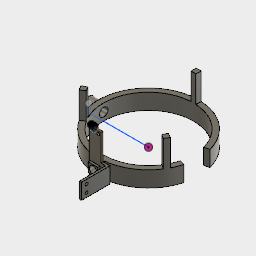
500 ml band v12 (Autodesk Fusion 360 design; units mm, degrees)
Autodesk Fusion 360 part; units mm, degrees
note: some values were not read from the file. Set by a fixed rule: which sketch regions a step uses.
sketch "Sketch1" plane through (0, 0, 0) normal (0, 1, 0) x (1, 0, 0)
  circle A0 centre (0, 0) radius 42.5
  circle A1 centre (0, 0) radius 47.5
  dimension "d1" = 85
  dimension "d2" = 5
  measures "d1" diameter of A0
extrude "Extrude1" add sketch "Sketch1" along normal blind 15
sketch "Sketch2" plane through (0, 15, 0) normal (0, 1, 0) x (-1, 0, 0)
  circle A0 centre (0, 0) radius 42.5
  circle A1 centre (0, 0) radius 47.5
  line L0 (0, 0) -> (2.4844, -47.435)
  line L1 (0, 0) -> (-2.5267, -47.4328)
extrude "Extrude2" add sketch "Sketch2" along normal blind 25 contours A0 A1 L0 L1 picked at (1.3425, -45.8073)
sketch "Sketch3" plane through (0, 15, 0) normal (0, 1, 0) x (-1, 0, 0)
  line L0 (2.2229, -42.4418) -> (2.4844, -47.435)
  arc A0 (2.4844, -47.435) -> (-2.5267, -47.4328) centre (0, 0) ccw
  line L1 (-2.5267, -47.4328) -> (-2.2607, -42.4398)
  arc A1 (2.2229, -42.4418) -> (-2.2607, -42.4398) centre (0, 0) ccw
  line L2 (0, 0) -> (42.3334, 21.5437)
  line L3 (0, 0) -> (39.8389, 25.8672)
extrude "Extrude3" add sketch "Sketch3" along normal blind 25 contours A0 A1 L2 L3
sketch "Sketch4" plane through (0, 15, 0) normal (0, 1, 0) x (-1, 0, 0)
  line L0 (35.6453, 23.1443) -> (39.8389, 25.8672)
  arc A0 (39.8389, 25.8672) -> (-2.5267, -47.4328) centre (0, 0) ccw
  line L1 (-2.5267, -47.4328) -> (-2.2607, -42.4398)
  arc A1 (35.6453, 23.1443) -> (-2.2607, -42.4398) centre (0, 0) ccw
  line L2 (0, 0) -> (-39.8369, 25.8704)
  line L3 (0, 0) -> (47.5, 0) construction
  line L4 (0, 0) -> (-42.3228, 21.5645)
  line L5 (0, 0) -> (47.5, 0) construction
  dimension "d9" = 147
  dimension "d10" = 47.5
  dimension "d11" = 153
  dimension "d12" = 47.5
  measures "d9" angle of L2 L3
  measures "d10" distance of A0.centre L2.end
  measures "d11" angle of L4 L5
  measures "d12" distance of A0.centre L4.end
extrude "Extrude4" add sketch "Sketch4" along normal blind 25 contours A0 A1 L2 L4
sketch "Sketch5" plane through (0, 15, 0) normal (0, 1, 0) x (-1, 0, 0)
  line L0 (-37.8678, 19.2946) -> (-42.3228, 21.5645)
  arc A0 (-42.3228, 21.5645) -> (-2.5267, -47.4328) centre (0, 0) ccw
  line L1 (-2.5267, -47.4328) -> (-2.2607, -42.4398)
  arc A1 (-37.8678, 19.2946) -> (-2.2607, -42.4398) centre (0, 0) ccw
  line L2 (0, 0) -> (-45.8815, 12.2939)
  line L3 (0, 0) -> (47.5, 0) construction
  line L4 (0, 0) -> (-45.8815, -12.2939)
  line L5 (0, 0) -> (47.5, 0) construction
  dimension "d15" = 165
  dimension "d16" = 47.5
  dimension "d17" = 165
  dimension "d18" = 47.5
  measures "d15" angle of L2 L3
  measures "d16" distance of A0.centre L2.end
  measures "d17" angle of L4 L5
  measures "d18" distance of A0.centre L4.end
extrude "Extrude5" cut sketch "Sketch5" against normal blind 15 contours A0 A1 L2 L4
sketch "Sketch6" plane through (0, 0, 0) normal (0, 0, 1) x (1, 0, 0)
  line L0 (0, 0) -> (5.5, 0)
  line L1 (5.5, 0) -> (5.5, 2)
  line L2 (5.5, 2) -> (-5.5, 2)
  line L3 (-5.5, 2) -> (-5.5, 13)
  line L4 (-5.5, 13) -> (5.5, 13)
  line L5 (5.5, 13) -> (5.5, 2)
  dimension "d21" = 5.5
  dimension "d22" = 2
  dimension "d23" = 11
  dimension "d24" = 11
  measures "d21" distance of L0.start L0.end
  measures "d22" distance of L0.end L1.end
  measures "d23" distance of L1.end L2.end
  measures "d24" distance of L1.end L4.end
extrude "Extrude6" cut sketch "Sketch6" along normal blind 50
sketch "Sketch8" plane through (0, 0, 0) normal (0, 0, 1) x (1, 0, 0)
  line L0 (0, 0) -> (-56.7, 0)
  line L1 (-56.7, 0) -> (-56.7, 7.5)
  dimension "d28" = 56.7
  dimension "d29" = 7.5
  measures "d28" distance of L0.start L0.end
  measures "d29" distance of L0.end L1.end
sketch "Sketch9" plane through (0, 0, 0) normal (1, 0, 0) x (0, 0, -1)
  point P0 (0, 7.5)
ref_plane "WorkPlane1" through (-56.7, 7.5, 0) normal (1, 0, 0) x (0, 0, -1)
cylinder "CylinderPrimitive1" add diameter 12 height 14.2 placed x (0, 0, -1) y (0, 1, 0) z (1, 0, 0) at (-56.7, 7.5, 0)
hole "Hole1" at (-56.7, 7.5, 0) direction (1, 0, 0) diameter 6.8 depth 2.2 tip angle 180
sketch "Sketch11" plane through (0, 0, 0) normal (1, 0, 0) x (0, 0, -1)
  circle A0 centre (0, 7.5) radius 4
  point P0 (0, 7.5)
  dimension "d37" = 8
  measures "d37" diameter of A0
extrude "Extrude7" cut sketch "Sketch11" against normal blind 54.5
sketch "Sketch16" plane through (0, 0, 0) normal (0, 1, 0) x (1, 0, 0)
extrude "Extrude13" add sketch "Sketch6" along normal blind 50.5
move_face "OffsetFaces2" offset -42.5 1 faces at (1.8333, 5.6667, 0)
sketch "Sketch17" plane through (0, 0, 50.5) normal (0, 0, 1) x (1, 0, 0)
  line L0 (5.5, 13) -> (-5.5, 13)
  line L1 (-5.5, 13) -> (-5.5, 2)
  line L2 (-5.5, 2) -> (5.5, 2)
  line L3 (5.5, 2) -> (5.5, 13)
  line L4 (-4.5, 12) -> (-4.5, 3)
  line L5 (-4.5, 3) -> (4.5, 3)
  line L6 (4.5, 3) -> (4.5, 12)
  line L7 (4.5, 12) -> (-4.5, 12)
  dimension "d60" = 1
extrude "Extrude14" add sketch "Sketch17" along normal blind 2 contours L4 L5 L6 L7
move_face "OffsetFaces3" offset 2 1 faces at (-0.6123, 13, 49.4882)
move_face "OffsetFaces4" offset 2 1 faces at (-0.6123, 2, 49.4882)
sketch "Sketch18" plane through (0, 0, 52.5) normal (0, 0, 1) x (1, 0, 0)
  line L0 (4.5, 12) -> (-4.5, 12)
  line L1 (-4.5, 12) -> (-4.5, 3)
  line L2 (-4.5, 3) -> (4.5, 3)
  line L3 (4.5, 3) -> (4.5, 12)
  line L4 (-4.5, 12) -> (0, 7.5)
  circle A0 centre (0, 7.5) radius 3.5
  circle A1 centre (0, 7.5) radius 2
  point P0 (0, 7.5)
  dimension "d65" = 7
  dimension "d66" = 4
  measures "d65" diameter of A0
  measures "d66" diameter of A1
extrude "Extrude15" cut sketch "Sketch18" against normal blind 11 contours A1
sketch "Sketch19" plane through (0, 0, 52.5) normal (0, 0, 1) x (1, 0, 0)
  circle A0 centre (0, 7.5) radius 2
  line L0 (4.5, 12) -> (-4.5, 12)
  line L1 (-4.5, 12) -> (-4.5, 3)
  line L2 (-4.5, 3) -> (4.5, 3)
  line L3 (4.5, 3) -> (4.5, 12)
  line L4 (-4.5, 12) -> (0, 7.5)
  circle A1 centre (0, 7.5) radius 3.5
  dimension "d69" = 7
  measures "d69" diameter of A1
extrude "Extrude16" cut sketch "Sketch19" against normal blind 9 contours A1
sketch "Sketch20" plane through (0, 15, 0) normal (0, 1, 0) x (-1, 0, 0)
  line L0 (-39.8369, 25.8704) -> (-35.6435, 23.1472)
  arc A0 (35.6453, 23.1443) -> (-35.6435, 23.1472) centre (0, 0) ccw
  line L1 (35.6453, 23.1443) -> (39.8389, 25.8672)
  arc A1 (39.8389, 25.8672) -> (5.5, 47.1805) centre (0, 0) ccw
  line L2 (5.5, 47.1805) -> (5.5, 50.5)
  line L3 (5.5, 50.5) -> (-5.5, 50.5)
  line L4 (-5.5, 50.5) -> (-5.5, 47.1805)
  arc A2 (-5.5, 47.1805) -> (-39.8369, 25.8704) centre (0, 0) ccw
  line L5 (5.5, 50.5) -> (-5.5, 50.5)
  line L6 (-5.5, 50.5) -> (-5.5, 48.5)
  line L7 (-5.5, 48.5) -> (5.5, 48.5)
  line L8 (5.5, 48.5) -> (5.5, 50.5)
  dimension "d72" = 2
  measures "d72" distance of L2.end L7.end
extrude "Extrude17" add sketch "Sketch20" along normal blind 25 contours L2 L3 L4 L5 L6 L7 L8
sketch "Sketch21" plane through (5.5, 0, 0) normal (1, 0, 0) x (0, 0, -1)
  line L0 (-47.1805, 0) -> (-47.1805, 15)
  line L1 (-47.1805, 15) -> (-48.5, 15)
  line L2 (-48.5, 15) -> (-48.5, 40)
  line L3 (-48.5, 40) -> (-50.5, 40)
  line L4 (-50.5, 40) -> (-50.5, 0)
  line L5 (-50.5, 0) -> (-47.1805, 0)
  line L6 (-50.5, 0) -> (-48.5, 0)
  line L7 (-48.5, 0) -> (-48.5, 15)
  line L8 (-48.5, 15) -> (-50.5, 15)
  line L9 (-50.5, 15) -> (-50.5, 0)
  dimension "d75" = 15
  dimension "d76" = 2
  measures "d75" distance of L4.end L8.end
  measures "d76" distance of L4.end L6.end
extrude "Extrude18" add sketch "Sketch21" along normal blind 6.5 contours L4 L5 L6 L7 L8 L9
sketch "Sketch22" plane through (0, 0, 50.5) normal (0, 0, 1) x (1, 0, 0)
  line L0 (4.5, 12) -> (4.5, 3)
  line L1 (4.5, 3) -> (-4.5, 3)
  line L2 (-4.5, 3) -> (-4.5, 12)
  line L3 (-4.5, 12) -> (4.5, 12)
  line L4 (-5.5, 40) -> (-5.5, 0)
  line L5 (-5.5, 0) -> (12, 0)
  line L6 (12, 0) -> (12, 15)
  line L7 (12, 15) -> (5.5, 15)
  line L8 (5.5, 15) -> (5.5, 40)
  line L9 (5.5, 40) -> (-5.5, 40)
  line L10 (12, 15) -> (10, 15)
  line L11 (10, 15) -> (10, 0)
  line L12 (10, 0) -> (12, 0)
  line L13 (12, 0) -> (12, 15)
extrude "Extrude19" add sketch "Sketch22" along normal blind 25 contours L5 L6 L7 L10 L11 L12 L13
sketch "Sketch25" plane through (0, 0, 48.5) normal (0, 0, -1) x (-1, 0, 0)
  line L0 (-5.5, 15) -> (5.5, 15)
  line L1 (5.5, 15) -> (5.5, 40)
  line L2 (5.5, 40) -> (-5.5, 40)
  line L3 (-5.5, 40) -> (-5.5, 15)
  line L4 (-5.5, 40) -> (-3, 40)
  line L5 (-3, 40) -> (-3, 37.5)
  circle A0 centre (-3, 37.5) radius 1.3
  dimension "d90" = 2.5
  dimension "d91" = 2.5
  dimension "d92" = 2.6
  measures "d90" distance of L2.end L4.end
  measures "d91" distance of L4.end L5.end
  measures "d92" diameter of A0
extrude "Extrude22" cut sketch "Sketch25" against normal blind 2 contours A0
sketch "Sketch26" plane through (0, 0, 48.5) normal (0, 0, -1) x (-1, 0, 0)
  circle A0 centre (-3, 37.5) radius 1.3
  line L0 (-5.5, 15) -> (5.5, 15)
  line L1 (5.5, 15) -> (5.5, 40)
  line L2 (5.5, 40) -> (-5.5, 40)
  line L3 (-5.5, 40) -> (-5.5, 15)
  line L4 (5.5, 40) -> (3, 40)
  line L5 (3, 40) -> (3, 37.5)
  circle A1 centre (3, 37.5) radius 1.3
  dimension "d95" = 2.5
  dimension "d96" = 2.5
  dimension "d97" = 2.6
  measures "d95" distance of L1.end L4.end
  measures "d96" distance of L4.end L5.end
  measures "d97" diameter of A1
extrude "Extrude23" cut sketch "Sketch26" against normal blind 2 contours A1
sketch "Sketch27" plane through (12, 0, 0) normal (1, 0, 0) x (0, 0, -1)
  line L0 (-75.5, 0) -> (-48.5, 0)
  line L1 (-48.5, 0) -> (-48.5, 15)
  line L2 (-48.5, 15) -> (-75.5, 15)
  line L3 (-75.5, 15) -> (-75.5, 0)
  line L4 (-75.5, 15) -> (-70.5, 15)
  line L5 (-70.5, 15) -> (-70.5, 11)
  circle A0 centre (-70.5, 11) radius 1.3
  dimension "d100" = 5
  dimension "d101" = 4
  dimension "d102" = 2.6
  measures "d100" distance of L2.end L4.end
  measures "d101" distance of L4.end L5.end
  measures "d102" diameter of A0
extrude "Extrude24" cut sketch "Sketch27" against normal blind 2 contours A0
sketch "Sketch28" plane through (12, 0, 0) normal (1, 0, 0) x (0, 0, -1)
  circle A0 centre (-70.5, 11) radius 1.3
  line L0 (-75.5, 0) -> (-48.5, 0)
  line L1 (-48.5, 0) -> (-48.5, 15)
  line L2 (-48.5, 15) -> (-75.5, 15)
  line L3 (-75.5, 15) -> (-75.5, 0)
  line L4 (-75.5, 0) -> (-70.5, 0)
  line L5 (-70.5, 0) -> (-70.5, 4)
  circle A1 centre (-70.5, 4) radius 1.3
  dimension "d105" = 5
  dimension "d106" = 4
  dimension "d107" = 2.6
  measures "d105" distance of L0.start L4.end
  measures "d106" distance of L4.end L5.end
  measures "d107" diameter of A1
extrude "Extrude25" cut sketch "Sketch28" against normal blind 2 contours A1
sketch "Sketch29" plane through (0, 0, 50.5) normal (0, 0, 1) x (1, 0, 0)
  circle A0 centre (-3, 37.5) radius 1.3
  circle A1 centre (3, 37.5) radius 1.3
  line L0 (10, 0) -> (10, 15)
  line L1 (10, 15) -> (5.5, 15)
  line L2 (5.5, 15) -> (5.5, 40)
  line L3 (5.5, 40) -> (-5.5, 40)
  line L4 (-5.5, 40) -> (-5.5, 0)
  line L5 (-5.5, 0) -> (10, 0)
  line L6 (4.5, 12) -> (4.5, 3)
  line L7 (4.5, 3) -> (-4.5, 3)
  line L8 (-4.5, 3) -> (-4.5, 12)
  line L9 (-4.5, 12) -> (4.5, 12)
